Autodesk Inventor part; units mm, degrees
(part 5 of 5)
  arc A2302 (-16.614, -14.2919) -> (-16.722, -14.4863) centre (-15.5907, -14.9875) ccw
  arc A2303 (-16.722, -14.4863) -> (-16.6833, -14.5457) centre (-16.6833, -14.5034) ccw
  arc A2304 (-16.6833, -14.5457) -> (-16.364, -14.4221) centre (-16.6833, -14.0714) ccw
  arc A2305 (-16.364, -14.4221) -> (-15.7284, -13.8044) centre (-25.5328, -4.3522) ccw
  arc A2306 (-15.7284, -13.8044) -> (-15.1286, -13.148) centre (-27.7148, -2.2486) ccw
  arc A2307 (-15.1286, -13.148) -> (-15.136, -12.9408) centre (-15.2436, -13.0484) ccw
  arc A2308 (-15.136, -12.9408) -> (-15.2228, -12.932) centre (-15.1848, -12.9895) ccw
  arc A2309 (-15.2228, -12.932) -> (-15.4687, -13.1078) centre (-12.9519, -16.3686) ccw
  arc A2310 (-15.4687, -13.1078) -> (-15.7663, -13.3595) centre (-12.8053, -16.5585) ccw
  arc A2311 (-15.7663, -13.3595) -> (-16.0961, -13.6818) centre (-9.9901, -19.6001) ccw
  arc A2312 (-8.394, -13.5401) -> (-8.765, -14.0544) centre (-6.9912, -14.9428) ccw
  arc A2313 (-8.765, -14.0544) -> (-8.8769, -14.5817) centre (-7.8107, -14.5324) ccw
  arc A2314 (-8.8769, -14.5817) -> (-8.7186, -15.1214) centre (-7.6904, -14.5268) ccw
  arc A2315 (-8.7186, -15.1214) -> (-8.2954, -15.6725) centre (-6.4085, -13.7855) ccw
  arc A2316 (-8.2954, -15.6725) -> (-7.8135, -16.0761) centre (-5.7719, -13.1489) ccw
  arc A2317 (-7.8135, -16.0761) -> (-7.3942, -16.2454) centre (-7.2343, -15.2456) ccw
  arc A2318 (-7.3942, -16.2454) -> (-6.9318, -16.2189) centre (-7.2235, -15.1778) ccw
  arc A2319 (-6.9318, -16.2189) -> (-6.3068, -15.9905) centre (-8.096, -12.0636) ccw
  arc A2320 (-6.3068, -15.9905) -> (-5.8185, -15.6226) centre (-6.8924, -14.7053) ccw
  arc A2321 (-5.8185, -15.6226) -> (-5.5333, -15.0839) centre (-6.8804, -14.7155) ccw
  arc A2322 (-5.5333, -15.0839) -> (-5.4965, -14.4513) centre (-7.0075, -14.6808) ccw
  arc A2323 (-5.4965, -14.4513) -> (-5.713, -13.8192) centre (-7.3479, -14.7325) ccw
  arc A2324 (-5.713, -13.8192) -> (-6.2117, -13.3188) centre (-6.8518, -14.4553) ccw
  arc A2325 (-6.2117, -13.3188) -> (-6.9584, -13.081) centre (-7.1581, -14.9992) ccw
  arc A2326 (-6.9584, -13.081) -> (-7.7556, -13.1573) centre (-7.1679, -15.0932) ccw
  arc A2327 (-7.7556, -13.1573) -> (-8.394, -13.5401) centre (-7.3105, -14.6235) ccw
  arc A2328 (-6.029, -13.969) -> (-6.4087, -13.5629) centre (-6.8166, -14.325) ccw
  arc A2329 (-5.9189, -14.5767) -> (-6.029, -13.969) centre (-7.1878, -14.4928) ccw
  arc A2330 (-6.1077, -15.2117) -> (-5.9189, -14.5767) centre (-7.4131, -14.4779) ccw
  arc A2331 (-6.549, -15.684) -> (-6.1077, -15.2117) centre (-7.2962, -14.5436) ccw
  arc A2332 (-6.9292, -15.9072) -> (-6.549, -15.684) centre (-9.0119, -11.9251) ccw
  arc A2333 (-7.1687, -15.9661) -> (-6.9292, -15.9072) centre (-7.1687, -15.4493) ccw
  arc A2334 (-7.4082, -15.9072) -> (-7.1687, -15.9661) centre (-7.1687, -15.4493) ccw
  arc A2335 (-7.7884, -15.684) -> (-7.4082, -15.9072) centre (-5.3255, -11.9251) ccw
  arc A2336 (-8.2008, -15.2689) -> (-7.7884, -15.684) centre (-7.0139, -14.5019) ccw
  arc A2337 (-8.392, -14.7361) -> (-8.2008, -15.2689) centre (-7.1547, -14.5929) ccw
  arc A2338 (-8.3266, -14.1792) -> (-8.392, -14.7361) centre (-7.1818, -14.596) ccw
  arc A2339 (-8.0186, -13.6958) -> (-8.3266, -14.1792) centre (-7.0821, -14.6323) ccw
  arc A2340 (-7.6679, -13.4348) -> (-8.0186, -13.6958) centre (-6.9535, -14.7609) ccw
  arc A2341 (-7.296, -13.3246) -> (-7.6679, -13.4348) centre (-7.218, -14.27) ccw
  arc A2342 (-6.8831, -13.3676) -> (-7.296, -13.3246) centre (-7.2037, -14.4426) ccw
  arc A2343 (-6.4087, -13.5629) -> (-6.8831, -13.3676) centre (-7.6118, -15.8109) ccw
  arc A2344 (21.9962, -13.5117) -> (21.6204, -14.3331) centre (23.1058, -14.5159) ccw
  arc A2345 (21.6204, -14.3331) -> (21.7576, -15.2721) centre (23.4017, -14.5523) ccw
  arc A2346 (21.7576, -15.2721) -> (22.3535, -16.0068) centre (23.3891, -14.5579) ccw
  arc A2347 (22.3535, -16.0068) -> (23.2084, -16.2809) centre (23.2084, -14.8107) ccw
  arc A2348 (23.2084, -16.2809) -> (23.7559, -16.143) centre (23.2084, -15.1256) ccw
  arc A2349 (23.7559, -16.143) -> (24.3865, -15.713) centre (22.0269, -12.9297) ccw
  arc A2350 (24.3865, -15.713) -> (24.8982, -15.1775) centre (22.0988, -13.0145) ccw
  arc A2351 (24.8982, -15.1775) -> (25.0563, -14.7143) centre (24.2988, -14.7143) ccw
  arc A2352 (25.0563, -14.7143) -> (25.0229, -14.5369) centre (24.5678, -14.7143) ccw
  arc A2353 (25.0229, -14.5369) -> (24.9054, -14.2755) centre (22.3944, -15.562) ccw
  arc A2354 (24.9054, -14.2755) -> (24.7392, -13.9873) centre (21.9149, -15.8076) ccw
  arc A2355 (24.7392, -13.9873) -> (24.5425, -13.7115) centre (21.7094, -15.9401) ccw
  arc A2356 (24.5425, -13.7115) -> (23.9875, -13.2561) centre (23.2327, -14.7419) ccw
  arc A2357 (23.9875, -13.2561) -> (23.2712, -13.0546) centre (23.1216, -14.9604) ccw
  arc A2358 (23.2712, -13.0546) -> (22.5545, -13.1446) centre (23.1312, -14.8388) ccw
  arc A2359 (22.5545, -13.1446) -> (21.9962, -13.5117) centre (22.9837, -14.4054) ccw
  arc A2360 (24.4962, -14.5242) -> (24.1797, -13.7921) centre (23.2605, -14.6239) ccw
  arc A2361 (24.3036, -15.3024) -> (24.4962, -14.5242) centre (23.2377, -14.6257) ccw
  arc A2362 (23.6761, -15.8191) -> (24.3036, -15.3024) centre (23.2003, -14.602) ccw
  arc A2363 (22.8627, -15.8667) -> (23.6761, -15.8191) centre (23.1962, -14.5915) ccw
  arc A2364 (22.2824, -15.3789) -> (22.8627, -15.8667) centre (23.0863, -15.0116) ccw
  arc A2365 (22.1385, -14.4745) -> (22.2824, -15.3789) centre (23.8394, -14.6676) ccw
  arc A2366 (22.4816, -13.6343) -> (22.1385, -14.4745) centre (23.8009, -14.6632) ccw
  arc A2367 (23.1534, -13.3063) -> (22.4816, -13.6343) centre (23.1534, -14.1582) ccw
  arc A2368 (23.4102, -13.3417) -> (23.1534, -13.3063) centre (23.1534, -14.2548) ccw
  arc A2369 (23.6969, -13.449) -> (23.4102, -13.3417) centre (22.9165, -15.0976) ccw
  arc A2370 (23.9683, -13.6061) -> (23.6969, -13.449) centre (22.885, -15.1641) ccw
  arc A2371 (24.1797, -13.7921) -> (23.9683, -13.6061) centre (23.2607, -14.6237) ccw
  point P0 (0, 0)
  point P1 (50.9531, -6.4169)
  point P2 (50.092, -5.8454)
  point P3 (48.6396, -5.6495)
  point P4 (43.5108, -5.6219)
  point P5 (39.7677, -5.6364)
  point P6 (37.8105, -5.6965)
  point P7 (36.5972, -5.8141)
  point P8 (35.8076, -6.0355)
  point P9 (34.5562, -6.3835)
  point P10 (32.9948, -6.4727)
  point P11 (31.4238, -6.3153)
  point P12 (30.1379, -5.9131)
  point P13 (27.0472, -3.259)
  point P14 (25.8897, 0.6063)
  point P15 (27.0344, 4.4484)
  point P16 (30.1113, 7.0505)
  point P17 (31.4161, 7.4463)
  point P18 (32.9982, 7.603)
  point P19 (34.5626, 7.5186)
  point P20 (35.8076, 7.1795)
  point P21 (36.598, 6.9626)
  point P22 (37.8327, 6.8468)
  point P23 (39.8156, 6.787)
  point P24 (43.5525, 6.7724)
  point P25 (51.1073, 7.8259)
  point P26 (51.8997, 9.0474)
  point P27 (52.1512, 9.8856)
  point P28 (52.0487, 10.8827)
  point P29 (51.4316, 12.9575)
  point P30 (50.503, 16.1693)
  point P31 (50.5853, 17.4879)
  point P32 (51.4074, 18.741)
  point P33 (55.2083, 22.4875)
  point P34 (57.1732, 24.3852)
  point P35 (58.9998, 26.1371)
  point P36 (60.5391, 27.603)
  point P37 (61.2015, 28.2131)
  point P38 (62.1894, 29.2632)
  point P39 (62.7285, 30.2629)
  point P40 (63.0404, 31.6852)
  point P41 (63.3115, 34.5551)
  point P42 (63.4931, 37.4258)
  point P43 (63.4137, 38.7986)
  point P44 (63.0608, 39.6824)
  point P45 (62.3323, 40.4645)
  point P46 (61.7943, 40.78)
  point P47 (61.2117, 40.9238)
  point P48 (60.2699, 40.951)
  point P49 (57.9038, 40.8625)
  point P50 (56.4262, 40.7914)
  point P51 (55.064, 40.7096)
  point P52 (53.9251, 40.6276)
  point P53 (53.4652, 40.5662)
  point P54 (52.6879, 40.2169)
  point P55 (51.3557, 39.1139)
  point P56 (49.183, 37.1068)
  point P57 (44.6444, 32.7271)
  point P58 (42.7401, 30.9041)
  point P59 (41.0144, 29.3026)
  point P60 (39.5441, 27.9774)
  point P61 (39.0671, 27.6446)
  point P62 (38.5752, 27.459)
  point P63 (37.7902, 27.3064)
  point P64 (36.762, 27.1823)
  point P65 (35.4674, 27.0905)
  point P66 (28.6511, 25.0045)
  point P67 (26.8555, 24.1315)
  point P68 (24.7324, 23.1025)
  point P69 (22.6258, 22.0839)
  point P70 (20.8812, 21.2432)
  point P71 (-4.1106, 20.9018)
  point P72 (-5.3285, 21.4718)
  point P73 (-6.4012, 21.9521)
  point P74 (-7.3202, 22.3478)
  point P75 (-7.5227, 22.3891)
  point P76 (-7.6663, 22.4146)
  point P77 (-7.8689, 22.5016)
  point P78 (-8.0891, 22.6255)
  point P79 (-8.2957, 22.7721)
  point P80 (-8.6618, 23.0111)
  point P81 (-10.2026, 23.8217)
  point P82 (-12.033, 24.7645)
  point P83 (-14.1096, 25.8088)
  point P84 (-16.9446, 27.2426)
  point P85 (-18.5176, 28.1127)
  point P86 (-19.4748, 28.7522)
  point P87 (-19.9972, 29.3053)
  point P88 (-20.4506, 30.16)
  point P89 (-20.7879, 31.1801)
  point P90 (-21.1773, 32.913)
  point P91 (-22.0448, 37.3862)
  point P92 (-22.4639, 39.5116)
  point P93 (-22.859, 41.3835)
  point P94 (-23.2124, 42.9637)
  point P95 (-23.3497, 43.3353)
  point P96 (-23.6158, 43.7396)
  point P97 (-23.9597, 44.0911)
  point P98 (-24.6294, 44.6303)
  point P99 (-27.2318, 46.6198)
  point P100 (-28.9487, 47.9049)
  point P101 (-29.8862, 48.5159)
  point P102 (-30.5636, 48.8127)
  point P103 (-31.2169, 48.9127)
  point P104 (-31.7218, 48.8755)
  point P105 (-32.1386, 48.7625)
  point P106 (-32.5186, 48.5551)
  point P107 (-32.9118, 48.231)
  point P108 (-33.7482, 47.2048)
  point P109 (-35.3625, 44.5463)
  point P110 (-36.924, 41.8255)
  point P111 (-37.3199, 40.7523)
  point P112 (-37.3294, 40.2564)
  point P113 (-36.8969, 37.6163)
  point P114 (-36.3581, 34.5397)
  point P115 (-35.6931, 31.0149)
  point P116 (-34.8694, 26.6834)
  point P117 (-34.3851, 23.8802)
  point P118 (-34.0925, 21.9108)
  point P119 (-34.155, 21.3608)
  point P120 (-34.3185, 21.062)
  point P121 (-34.6814, 20.6027)
  point P122 (-35.1373, 20.0934)
  point P123 (-35.6353, 19.6)
  point P124 (-47.0034, 18.4056)
  point P125 (-51.1447, 18.4014)
  point P126 (-55.2197, 18.4031)
  point P127 (-58.7387, 18.4096)
  point P128 (-60.7691, 18.4215)
  point P129 (-63.1356, 18.4303)
  point P130 (-64.0239, 18.3685)
  point P131 (-64.5589, 18.193)
  point P132 (-65.0451, 17.8304)
  point P133 (-65.3966, 17.3849)
  point P134 (-65.5766, 16.9262)
  point P135 (-65.6529, 16.2301)
  point P136 (-65.6695, 14.6996)
  point P137 (-65.6518, 13.7068)
  point P138 (-65.5983, 12.7955)
  point P139 (-65.5226, 12.0428)
  point P140 (-65.4277, 11.7416)
  point P141 (-65.2326, 11.5002)
  point P142 (-64.683, 11.0546)
  point P143 (-63.996, 10.5482)
  point P144 (-63.2287, 10.0344)
  point P145 (-62.3944, 9.4689)
  point P146 (-61.7482, 8.9601)
  point P147 (-61.2933, 8.5231)
  point P148 (-61.1189, 8.2094)
  point P149 (-60.9236, 6.7099)
  point P150 (-60.9654, 0.2597)
  point P151 (-61.0492, -6.4223)
  point P152 (-61.2783, -7.2762)
  point P153 (-61.5015, -7.5553)
  point P154 (-62.0441, -8.0177)
  point P155 (-62.7195, -8.5338)
  point P156 (-63.4625, -9.0436)
  point P157 (-64.1955, -9.5449)
  point P158 (-64.8377, -10.0333)
  point P159 (-65.3508, -10.4676)
  point P160 (-65.5076, -10.694)
  point P161 (-65.5713, -10.9747)
  point P162 (-65.6219, -11.7177)
  point P163 (-65.6576, -12.609)
  point P164 (-65.6695, -13.5856)
  point P165 (-65.6527, -15.0785)
  point P166 (-65.5769, -15.7726)
  point P167 (-65.4007, -16.2293)
  point P168 (-65.061, -16.664)
  point P169 (-35.56, -18.5257)
  point P170 (-35.0417, -19.0492)
  point P171 (-34.5802, -19.5857)
  point P172 (-34.2239, -20.0672)
  point P173 (-34.0855, -20.3742)
  point P174 (-34.0594, -21.0488)
  point P175 (-34.6127, -24.2087)
  point P176 (-35.4855, -28.8682)
  point P177 (-37.0712, -36.9536)
  point P178 (-37.2096, -37.7513)
  point P179 (-37.3057, -38.5299)
  point P180 (-37.3541, -39.1971)
  point P181 (-37.3261, -39.5707)
  point P182 (-36.9138, -40.6825)
  point P183 (-35.2402, -43.5792)
  point P184 (-33.5006, -46.4468)
  point P185 (-32.7638, -47.2701)
  point P186 (-32.1559, -47.5931)
  point P187 (-31.38, -47.7432)
  point P188 (-30.579, -47.7064)
  point P189 (-29.8958, -47.4767)
  point P190 (-29.5663, -47.2708)
  point P191 (-28.7959, -46.6994)
  point P192 (-27.8869, -46.0031)
  point P193 (-26.9121, -45.232)
  point P194 (-25.9442, -44.4614)
  point P195 (-25.0535, -43.7647)
  point P196 (-24.304, -43.1885)
  point P197 (-24.0171, -42.9901)
  point P198 (-23.5257, -42.4562)
  point P199 (-23.1456, -41.4944)
  dimension "d2" = 130.09
  constraints: 4746 point on circle, 2372 centre point, 200 end point
  measures "d2" horizontal distance of point (-66.161, -14.456) point (63.929, -37.224)
extrude "Extrusion1" add sketch "Sketch1" along normal blind 3 contours A249 A250 A251 A252 A253 A254 A255 A256 A257 A258 A259 A260 A261 A262 A263 A264 A265 A266 A267 A268 A269 A270 A271 A272 A273 A274 A275 L22 L23 L24 L25 A276 A277 A278 A279 L26 L27 A280 A281 A282 A283 A284 A285 A286 A287 A288 A289 A290 A291 A292 A293 A294 A295 A296 A297 A298 A299 A300 A301 A302 A303 A304 A305 A306 A307 A308 A309 A310 A311 A312 A313 A314 A315 A316 A317 A318 A319 L28 L29 A320 A321 A322 A323 A324 A325 A326 A327 A328 A329 A330 A331 A332 A333 A334 A335 A336 A337 A338 A339 A340 A341 A342 A343 L30 L31 A344 A345 A346 A347 A348 A349 A350 A351 A352 A353 A354 A355 A356 A357 A358 A359 A360 A361 A362 A363 A364 A365 A366 A367 A368 A369 A370 A371 A372 A373 A374 A375 A376 A377 A378 A379 A380 A381 A382 A383 L32 L33 L34 L35 L36 L37 A384 A385 A386 A387 A388 A389 A390 A391 A392 A393 A394 A395 A396 A397 A398 A399 A400 A401 A402 A403 A404 A405 A406 A407 A408 A409 A410 A411 A412 A413 A414 A415 A416 A417 A418 A419 A420 A421 A422 A423 L38 L39 L40 L41 A424 A425 A426 A427 A428 A429 A430 A431 A432 A433 A434 A435 A436 A437 A438 A439 A440 A441 A442 A443 A444 A445 A446 A447 A448 A449 A450 A451 A452 A453 A454 A455 A456 A457 A458 A459 A460 A461 A462 A463 A464 A465 A466 A467 L42 L43 A468 A469 A470 A471 A472 A473 A474 A475 A476 A477 A478 A479 A480 A481 A482 A483 A484 A485 A486 A487 A488 A489 A490 A491 A248
sketch "Sketch2" plane through (0, 3, 0) normal (0, 1, 0) x (1, 0, 0)
  circle A0 centre (-23.6086, 14.5288) radius 4.9273
  circle A1 centre (6.6771, 14.5288) radius 4.6599
  circle A2 centre (6.6771, -16.1286) radius 5.0518
  circle A3 centre (-23.6086, -16.1286) radius 5.1742
  point P0 (0, 0)
  constraints: 4 centre point
extrude "Extrusion2" add sketch "Sketch2" against normal blind 3
sketch "Sketch3" plane through (0, 3, 0) normal (0, 1, 0) x (1, 0, 0)
  circle A0 centre (-23.2436, 14.6296) radius 1.6
  circle A1 centre (7.2564, 14.6296) radius 1.6
  circle A2 centre (7.6901, -15.8704) radius 1.6
  circle A3 centre (-22.8099, -15.8704) radius 1.6
  arc A4 (-25.8897, -0.6058) -> (-27.0473, 3.2592) centre (-32.9695, -0.6204) ccw projected
  line L0 (-32.9695, -0.6204) -> (10.6901, -0.6204)
  line L1 (-15.6666, -0.6204) -> (-0.3205, -0.6204)
  line L2 (-7.9936, -0.6204) -> (-7.9936, 21.9698)
  line L3 (-7.9936, -0.6204) -> (7.2564, -0.6204)
  point P0 (0, 0)
  dimension "d5" = 3.2
  dimension "d6" = 3.2
  dimension "d7" = 3.2
  dimension "d8" = 3.2
  dimension "d9" = 30.5
  dimension "d10" = 30.5
  dimension "d11" = 30.5
  dimension "d12" = 30.5
  dimension "d13" = 15.25
  dimension "d14" = 15.25
  dimension "d17" = 90
  dimension "d18" = 15.25
  dimension "d19" = 15.25
  dimension "d20" = 15.25
  constraints: 8 end point, 4 centre point, 3 point on line, 1 horizontal, 1 midpoint, 1 vertical
  measures "d5" diameter of A0
  measures "d6" diameter of A1
  measures "d7" diameter of A2
  measures "d8" diameter of A3
  measures "d9" distance of A1.centre A0.centre
  measures "d10" vertical distance of A3.centre A0.centre
  measures "d11" distance of A2.centre A3.centre
  measures "d12" vertical distance of A1.centre A2.centre
  measures "d13" distance from line of A0.centre L0
  measures "d14" distance from line of A1.centre L0
  measures "d17" angle of L0 L2
  measures "d18" distance of L2.start L3.end
  measures "d19" distance from line of L3.end L2
  measures "d20" distance from line of A1.centre L2
extrude "Extrusion3" cut sketch "Sketch3" against normal blind 3
sketch "Sketch4" plane through (0, 3, 0) normal (0, 1, 0) x (1, 0, 0)
  circle A0 centre (29.8495, 38.2698) radius 1.5
  circle A1 centre (-55.9919, 32.2964) radius 1.5
  circle A2 centre (-55.9919, -33.39) radius 1.5
  point P0 (0, 0)
  dimension "d23" = 3
  dimension "d24" = 3
  dimension "d25" = 3
  constraints: 3 centre point
  measures "d23" diameter of A0
  measures "d24" diameter of A1
  measures "d25" diameter of A2
extrude "Extrusion4" cut sketch "Sketch4" against normal blind 3
sketch "Sketch5" plane through (0, 3, 0) normal (0, 1, 0) x (1, 0, 0)
  arc A0 (31.3101, 37.9283) -> (31.3401, 38.4374) centre (29.8495, 38.2698) ccw projected
  circle A1 centre (29.8495, 38.2698) radius 1.5
  arc A2 (-54.5163, 32.0268) -> (-54.5234, 32.6024) centre (-55.9919, 32.2964) ccw projected
  circle A3 centre (-55.9919, 32.2964) radius 1.5
  arc A4 (-54.5453, -33.7867) -> (-54.495, -33.2937) centre (-55.9919, -33.39) ccw projected
  circle A5 centre (-55.9919, -33.39) radius 1.5
  circle A6 centre (-55.9919, -33.39) radius 4.0652
  circle A7 centre (-55.9919, 32.2964) radius 3.7909
  circle A8 centre (29.8495, 38.2698) radius 4.0357
  arc A9 (-30.1113, -7.0505) -> (-27.0344, -4.4484) centre (-32.9692, -0.5508) ccw projected
  line L0 (-32.9692, -0.5508) -> (85.1514, -0.5508)
  arc A10 (31.3401, -39.5391) -> (31.3101, -39.03) centre (29.8495, -39.3715) ccw
  circle A11 centre (29.8495, -39.3715) radius 1.5
  circle A12 centre (29.8495, -39.3715) radius 4.0357
  point P0 (0, 0)
  point P1 (-54.5234, 32.6024)
  point P2 (31.3401, 38.4374)
  point P3 (-54.495, -33.2937)
  constraints: 9 centre point, 8 coincident, 5 symmetric about line, 2 end point, 2 point on circle, 1 horizontal, 3 other
extrude "Extrusion5" add sketch "Sketch5" against normal blind 3
sketch "Sketch6" plane through (0, 3, 0) normal (0, 1, 0) x (1, 0, 0)
  arc A0 (-27.0344, -4.4484) -> (-25.8897, -0.6058) centre (-32.8637, -0.6201) ccw projected
  line L0 (-32.8637, -0.6201) -> (101.6053, -0.6201)
  circle A1 centre (-47.7405, 9.4799) radius 1.5
  circle A2 centre (-47.7405, -10.7202) radius 1.5
  circle A3 centre (-47.7405, 9.4799) radius 2.5
  circle A4 centre (-47.7405, -10.7202) radius 2.5
  line L1 (-43.5524, -6.7724) -> (-50.3374, -6.7724) projected
  arc A5 (-48.6396, 5.6495) -> (-43.5108, 5.6219) centre (-43.5104, 481.9367) ccw projected
  line L2 (-48.6396, 5.6495) -> (-43.5108, 5.6219)
  point P0 (0, 0)
  point P1 (-46.9449, -6.7724)
  dimension "d31" = 3
  dimension "d32" = 5
  dimension "d33" = 5
  dimension "d38" = 3.9478
  dimension "d39" = 3.8352
  constraints: 4 centre point, 4 end point, 2 coincident, 1 horizontal, 1 midpoint, 1 symmetric about line, 1 other
  measures "d31" diameter of A1
  measures "d32" diameter of A3
  measures "d33" diameter of A4
  measures "d38" vertical distance of point (-46.945, -6.772) A2.centre
  measures "d39" distance from line of L2 A1.centre
extrude "Extrusion6" add sketch "Sketch6" against normal blind 3 contours A3 | A4
sketch "Sketch7" plane through (0, 3, 0) normal (0, 1, 0) x (1, 0, 0)
  arc A0 (-46.7804, -11.8727) -> (-49.1973, -11.0777) centre (-47.7405, -10.7202) ccw projected
  circle A1 centre (-47.7405, -10.7202) radius 1.5
  point P0 (0, 0)
  point P1 (-49.1973, -11.0777)
  constraints: 1 centre point, 1 coincident
extrude "Extrusion7" cut sketch "Sketch7" against normal blind 3
sketch "Sketch8" plane through (0, 3, 0) normal (0, 1, 0) x (1, 0, 0)
  line L0 (17.2292, 11.9933) -> (18.6119, 7.4214)
  line L1 (18.6119, 7.4214) -> (20.9091, 5.9717)
  line L2 (20.9091, 5.9717) -> (27.6415, 12.1528)
  line L3 (26.4888, 13.4084) -> (28.7346, 10.9622) projected
  arc A0 (26.1413, 13.6754) -> (24.322, 15.5252) centre (-95.7981, -104.4298) ccw projected
  line L4 (25.34, 14.4971) -> (18.2939, 10.9088)
  line L5 (25.34, 14.4971) -> (27.6415, 12.1528)
  line L6 (17.2292, 11.9933) -> (24.322, 15.5252)
  line L7 (18.2939, 10.9088) -> (19.1309, 12.9403)
  point P0 (0, 0)
  constraints: 14 end point, 2 point on line, 1 point on circle, 1 tangent
extrude "Extrusion8" cut sketch "Sketch8" against normal blind 3 contours L6 L7 L4 L5 L2 L1 L0
sketch "Sketch9" plane through (0, 3, 0) normal (0, 1, 0) x (1, 0, 0)
  arc A0 (-27.0344, -4.4484) -> (-25.8897, -0.6058) centre (-32.8637, -0.6201) ccw projected
  line L0 (-32.8637, -0.6201) -> (88.4587, -0.6201)
  circle A1 centre (59.9231, -14.6201) radius 1.5
  circle A2 centre (59.9231, 13.3799) radius 1.5
  circle A3 centre (37.0306, 9.3799) radius 1.5
  circle A4 centre (37.0306, -10.6201) radius 1.5
  circle A5 centre (37.0306, 9.3799) radius 4.2001
  circle A6 centre (59.9231, 13.3799) radius 2.8139
  circle A7 centre (59.9231, -14.6201) radius 3.1887
  circle A8 centre (37.0306, -10.6201) radius 3.5086
  point P0 (0, 0)
  dimension "d42" = 3
  dimension "d43" = 3
  dimension "d44" = 3
  dimension "d45" = 3
  dimension "d46" = 14
  dimension "d47" = 14
  dimension "d48" = 10
  dimension "d49" = 10
  dimension "d50" = 22.8925
  constraints: 8 centre point, 4 coincident, 2 end point, 1 horizontal
  measures "d42" diameter of A1
  measures "d43" diameter of A2
  measures "d44" diameter of A3
  measures "d45" diameter of A4
  measures "d46" distance from line of A2.centre L0
  measures "d47" distance from line of L0 A1.centre
  measures "d48" distance from line of L0 A3.centre
  measures "d49" distance from line of L0 A4.centre
  measures "d50" horizontal distance of A2.centre A3.centre
extrude "Extrusion9" add sketch "Sketch9" against normal blind 3
sketch "Sketch10" plane through (0, 3, 0) normal (0, 1, 0) x (1, 0, 0)
  arc A0 (59.6137, -16.0879) -> (58.9632, -15.7728) centre (59.9231, -14.6201) ccw projected
  circle A1 centre (59.9231, -14.6201) radius 1.5
  point P0 (0, 0)
  point P1 (58.9632, -15.7728)
  point P2 (59.6137, -16.0879)
  constraints: 1 centre point, 1 coincident
extrude "Extrusion10" cut sketch "Sketch10" against normal blind 3
sketch "Sketch11" plane through (0, 3, 0) normal (0, 1, 0) x (1, 0, 0)
  circle A0 centre (53.4541, -0.5633) radius 2
  circle A1 centre (53.4541, -0.5633) radius 4.9271
  point P0 (0, 0)
  dimension "d55" = 4
  constraints: 2 centre point, 1 coincident
  measures "d55" diameter of A0
extrude "Extrusion11" add sketch "Sketch11" against normal blind 3
sketch "Sketch12" plane through (0, 3, 0) normal (0, 1, 0) x (1, 0, 0)
  circle A0 centre (50.9743, 12.0462) radius 2.3423
  circle A1 centre (46.9866, 4.4135) radius 2.5247
  circle A2 centre (47.1514, -5.6618) radius 3.8714
  circle A3 centre (51.2732, -13.4167) radius 2.3203
  point P0 (0, 0)
  constraints: 4 centre point
extrude "Extrusion12" add sketch "Sketch12" against normal blind 3
sketch "Sketch13" plane through (0, 3, 0) normal (0, 1, 0) x (1, 0, 0)
  arc A0 (-30.1113, -7.0505) -> (-27.0344, -4.4484) centre (-32.9692, -0.5508) ccw projected
  line L0 (-32.9692, -0.5508) -> (82.6738, -0.5508)
  circle A1 centre (47.0233, 4.4492) radius 1.05
  arc A2 (61.0492, 6.4223) -> (60.9654, -0.2597) centre (1550.8386, -15.5871) ccw projected
  line L1 (61.0492, 6.4223) -> (60.9654, -0.2597)
  circle A3 centre (51.0233, 12.4492) radius 1.05
  circle A4 centre (47.0233, -5.5508) radius 1.05
  circle A5 centre (51.0233, -13.5508) radius 1.05
  point P0 (0, 0)
  dimension "d60" = 2.1
  dimension "d61" = 5
  dimension "d62" = 14
  dimension "d63" = 2.1
  dimension "d64" = 8
  dimension "d65" = 4
  constraints: 4 centre point, 4 end point, 2 symmetric about line, 1 horizontal, 2 other
  measures "d60" diameter of A1
  measures "d61" distance from line of L0 A1.centre
  measures "d62" distance from line of L1 A1.centre
  measures "d63" diameter of A3
  measures "d64" vertical distance of A3.centre A1.centre
  measures "d65" horizontal distance of A1.centre A3.centre
extrude "Extrusion13" cut sketch "Sketch13" against normal blind 3 contours A1 | A3 | A4 | A5
sketch "Sketch14" plane through (0, 3, 0) normal (0, 1, 0) x (1, 0, 0)
  circle A0 centre (-22.8099, -15.8704) radius 1.6 projected
  circle A1 centre (7.2564, 14.6296) radius 1.6 projected
  line L0 (-22.8099, -15.8704) -> (7.2564, 14.6296)
  circle A2 centre (-23.2436, 14.6296) radius 1.6 projected
  circle A3 centre (7.6901, -15.8704) radius 1.6 projected
  line L1 (-23.2436, 14.6296) -> (7.6901, -15.8704)
  circle A4 centre (-23.2436, 14.6296) radius 2.5
  circle A5 centre (7.2564, 14.6296) radius 2.5
  circle A6 centre (7.6901, -15.8704) radius 2.5
  circle A7 centre (-22.8099, -15.8704) radius 2.5
  circle A8 centre (-23.2436, 14.6296) radius 1.6
  circle A9 centre (7.2564, 14.6296) radius 1.6
  circle A10 centre (7.6901, -15.8704) radius 1.6
  circle A11 centre (-22.8099, -15.8704) radius 1.6
  circle A12 centre (-23.2436, 14.6296) radius 1.6
  circle A13 centre (7.2564, 14.6296) radius 1.6
  circle A14 centre (7.6901, -15.8704) radius 1.6
  circle A15 centre (-22.8099, -15.8704) radius 1.5
  point P0 (0, 0)
  dimension "d68" = 5
  dimension "d69" = 5
  dimension "d70" = 5
  dimension "d71" = 5
  constraints: 12 centre point, 11 coincident, 7 concentric, 4 end point, 1 point on line
  measures "d68" diameter of A4
  measures "d69" diameter of A5
  measures "d70" diameter of A6
  measures "d71" diameter of A7
extrude "Extrusion14" add sketch "Sketch14" along normal blind 1 contours A7 | A4 | A5 | A6
sketch "Sketch15" plane through (0, 3, 0) normal (0, 1, 0) x (1, 0, 0)
  circle A0 centre (-23.2436, 14.6296) radius 1.6 projected
  circle A1 centre (7.6901, -15.8704) radius 1.6 projected
  line L0 (-23.2436, 14.6296) -> (7.6901, -15.8704)
  circle A2 centre (-22.8099, -15.8704) radius 1.6 projected
  circle A3 centre (7.2564, 14.6296) radius 1.6 projected
  line L1 (-22.8099, -15.8704) -> (7.2564, 14.6296)
  line L2 (-7.7767, -0.6204) -> (-7.7767, 19.3796)
  line L3 (-7.7767, 19.3796) -> (3.7233, 19.3796)
  line L4 (3.7233, 19.3796) -> (3.7233, -20.6204)
  line L5 (3.7233, -20.6204) -> (-19.2767, -20.6204)
  line L6 (-19.2767, -20.6204) -> (-19.2767, 19.3796)
  line L7 (-19.2767, 19.3796) -> (-7.7767, 19.3796)
  point P0 (0, 0)
  dimension "d74" = 20
  dimension "d75" = 11.5
  dimension "d76" = 40
  dimension "d77" = 23
  constraints: 16 end point, 4 perpendicular, 1 horizontal, 1 midpoint, 1 vertical
  measures "d74" distance of L2.start L2.end
  measures "d75" distance of L2.end L3.end
  measures "d76" distance of L3.end L4.end
  measures "d77" distance of L4.end L5.end
extrude "Extrusion15" cut sketch "Sketch15" against normal blind 0.5 contours L6 L7 L2 L0 | L0 L1 L6 | L1 L4 L0 | L0 L4 L5 L6 L1 | L2 L3 L4 L1
sketch "Sketch17" plane through (0, 2.5, 0) normal (0, 1, 0) x (1, 0, 0)
  arc A0 (-27.0344, -4.4484) -> (-25.8897, -0.6058) centre (-32.8637, -0.6201) ccw projected
  line L0 (-32.8637, -0.6201) -> (36.5369, -0.6201)
  line L1 (-19.2767, -20.4716) -> (-19.2767, 19.3308) projected
  line L2 (-19.2767, -0.5704) -> (-17.2774, -0.6201)
  line L3 (-17.0783, -19.4145) -> (0.9872, -19.4145) projected
  line L4 (-17.2774, -0.6201) -> (-17.0783, -19.4145)
  line L5 (-19.2767, 19.3308) -> (-17.075, 18.264) projected
  line L6 (-17.2774, -0.6201) -> (-17.075, 18.264)
  line L7 (3.7233, 19.3796) -> (3.7233, -20.6204) projected
  line L8 (3.7233, -0.6204) -> (1.7233, -0.6201)
  line L9 (1.7233, -0.6201) -> (1.7253, 18.6194)
  line L10 (0.9918, 18.264) -> (3.2943, 19.3796) projected
  line L11 (1.7233, -0.6201) -> (1.7233, -19.765)
  line L12 (3.5196, -20.6204) -> (0.9872, -19.4145) projected
  line L13 (-17.075, 18.264) -> (1.728, 44.6098)
  line L14 (1.728, 44.6098) -> (1.7253, 18.6194)
  line L15 (1.7233, -19.765) -> (1.7195, -36.2978)
  line L16 (1.7195, -36.2978) -> (-17.0783, -19.4145)
  point P0 (0, 0)
  dimension "d80" = 2
  dimension "d81" = 2
  constraints: 22 end point, 4 point on line, 2 midpoint, 1 horizontal, 1 perpendicular, 1 vertical
  measures "d80" distance of L2.start L2.end
  measures "d81" distance of L8.start L8.end
extrude "Extrusion16" cut sketch "Sketch17" against normal blind 1.5 contours L6 L13 L14 L9 L0 | L0 L11 L12 L3 L4 | L3 L12 L15 L16
sketch "Sketch23" plane through (0, 3, 0) normal (0, 1, 0) x (1, 0, 0)
  line L0 (3.5196, -20.6204) -> (4.1106, -20.9018) projected
  line L1 (3.7291, -20.7201) -> (-8.0702, -20.7201)
  line L2 (-8.0702, -20.7201) -> (-8.0702, 34.9354)
  line L3 (-8.0702, 34.9354) -> (3.7291, 34.9354)
  line L4 (3.7291, 34.9354) -> (3.7291, -20.7201)
  point P0 (0, 0)
  constraints: 8 end point, 2 parallel, 1 horizontal, 1 perpendicular, 1 point on line
extrude "Extrusion22" cut sketch "Sketch23" against normal blind 0.5
sketch "Sketch25" plane through (0, 3, 0) normal (0, 1, 0) x (1, 0, 0)
  line L0 (-17.0783, -19.4145) -> (-19.2767, -20.4716) projected
  line L1 (9.9588, 22.6088) -> (0.9918, 18.264) projected
  line L2 (-17.0783, -19.4145) -> (0.9918, -19.4145)
  line L3 (0.9918, -19.4145) -> (0.9918, 18.264)
  line L4 (0.9918, 18.264) -> (-17.0783, 18.264)
  line L5 (-17.0783, 18.264) -> (-17.0783, -19.4145)
  line L6 (0.9918, 18.264) -> (3.7291, 19.5903)
  line L7 (3.7291, 19.5903) -> (3.7291, -20.7201) projected
  line L8 (3.7291, 19.5903) -> (3.7291, -20.7201)
  line L9 (3.7291, -20.7201) -> (0.9918, -19.4145)
  line L10 (-17.0783, -19.4145) -> (-19.2767, -20.4716)
  line L11 (-19.2767, -20.4716) -> (-19.2767, 19.3308) projected
  line L12 (-19.2767, -20.4716) -> (-19.2767, 19.3308)
  line L13 (-19.2767, 19.3308) -> (-17.0783, 18.264)
  point P0 (0, 0)
  constraints: 20 end point, 3 equal length, 1 horizontal, 1 perpendicular, 1 point on line, 1 vertical
extrude "Extrusion24" add sketch "Sketch25" against normal blind 3
sketch "Sketch26" plane through (0, 3, 0) normal (0, 1, 0) x (1, 0, 0)
  arc A0 (22.7174, 39.7245) -> (21.9043, 35.5673) centre (511.1801, -57.9702) ccw projected
  line L0 (21.9043, 35.5673) -> (50.154, 183.336)
  arc A1 (37.0712, 36.9536) -> (35.4855, 28.8679) centre (2745.9567, -498.4883) ccw projected
  line L1 (35.4855, 28.8679) -> (64.9873, 180.4994)
  circle A2 centre (57.8174, 183.336) radius 7.7106
  line L2 (21.9043, 35.5673) -> (35.4855, 28.8679)
  arc A3 (-30.1113, -7.0505) -> (-27.0344, -4.4484) centre (-32.9692, -0.5508) ccw projected
  line L3 (-32.9692, -0.5508) -> (-8.5446, -0.5508)
  arc A4 (21.9043, -36.669) -> (22.7174, -40.8262) centre (511.1801, 56.8685) ccw
  line L4 (21.9043, -36.669) -> (50.154, -184.4377)
  arc A5 (35.4855, -29.9696) -> (37.0712, -38.0553) centre (2745.9567, 497.3866) ccw
  line L5 (35.4855, -29.9696) -> (64.9873, -181.6011)
  circle A6 centre (57.8174, -184.4377) radius 7.7106
  line L6 (21.9043, -36.669) -> (35.4855, -29.9696)
  arc A7 (-47.8615, 34.6906) -> (-43.2688, 30.2663) centre (1782.7173, 1930.371) ccw projected
  line L7 (-43.2688, 30.2663) -> (-161.509, 151.4367)
  arc A8 (-52.5304, 18.7828) -> (-58.694, 24.7351) centre (-3130.1027, -3161.8952) ccw projected
  line L8 (-52.5304, 18.7828) -> (-171.9931, 141.2061)
  line L9 (-171.9931, 141.2061) -> (-161.509, 151.4367)
  circle A9 centre (-166.751, 146.3214) radius 7.3243
  line L10 (-52.5304, 18.7828) -> (-43.2688, 30.2663)
  arc A10 (-43.2688, 30.2663) -> (-41.045, 28.1667) centre (76.8371, 155.2473) ccw projected
  arc A11 (-43.2688, -31.368) -> (-47.8615, -35.7923) centre (1782.7173, -1931.4727) ccw
  line L11 (-43.2688, -31.368) -> (-161.509, -152.5384)
  arc A12 (-58.694, -25.8368) -> (-52.5304, -19.8845) centre (-3130.1027, 3160.7935) ccw
  line L12 (-52.5304, -19.8845) -> (-171.9931, -142.3078)
  line L13 (-171.9931, -142.3078) -> (-161.509, -152.5384)
  circle A13 centre (-166.751, -147.4231) radius 7.3243
  line L14 (-52.5304, -19.8845) -> (-43.2688, -31.368)
  arc A14 (-41.045, -29.2684) -> (-43.2688, -31.368) centre (76.8371, -156.349) ccw
  point P0 (0, 0)
  point P1 (50.1102, 183.1069)
  point P2 (50.1102, -184.2086)
  point P3 (-171.9931, 141.2061)
  constraints: 30 end point, 22 symmetric about line, 14 point on circle, 5 centre point, 3 horizontal, 2 point on line, 2 tangent, 1 midpoint, 1 parallel, 17 other
extrude "Extrusion25" add sketch "Sketch26" against normal blind 3
sketch "Sketch27" plane through (0, 3, 0) normal (0, 1, 0) x (1, 0, 0)
  line L0 (2.5588, 7.6763) -> (14.7911, 16.4959)
  line L1 (14.7911, 16.4959) -> (26.1866, 23.029)
  line L2 (26.1866, 23.029) -> (31.7397, 7.6763)
  line L3 (31.7397, 7.6763) -> (31.7397, -17.8026)
  line L4 (31.7397, -17.8026) -> (20.4889, -25.9145)
  line L5 (20.4889, -25.9145) -> (9.9183, -11.2536)
  line L6 (9.9183, -11.2536) -> (0.7077, -9.7451)
  line L7 (0.7077, -9.7451) -> (2.5588, 7.6763)
  line L8 (-42.9641, 19.7461) -> (-27.8918, 15.4972)
  line L9 (-27.8918, 15.4972) -> (-24.9576, 4.8081)
  line L10 (-24.9576, 4.8081) -> (-21.4242, -8.0633)
  line L11 (-21.4242, -8.0633) -> (-31.9676, -20.8613)
  line L12 (-31.9676, -20.8613) -> (-41.2126, -21.8585)
  line L13 (-41.2126, -21.8585) -> (-42.5193, -9.7451)
  line L14 (-43.5524, -6.7724) -> (-50.3374, -6.7724) projected
  line L15 (-42.5193, -9.7451) -> (-50.3374, -6.7724)
  arc A0 (-50.9531, 6.4169) -> (-50.092, 5.8454) centre (-49.6841, 7.3946) ccw projected
  line L16 (-50.3374, -6.7724) -> (-50.092, 5.8454)
  line L17 (-50.092, 5.8454) -> (-45.0482, 7.23)
  line L18 (-45.0482, 7.23) -> (-42.9641, 19.7461)
  line L19 (-51.6087, 11.162) -> (-52.3994, 8.8937) projected
  line L20 (-52.3994, 8.8937) -> (-52.1512, -9.8856)
  line L21 (-52.1512, -9.8856) -> (-50.3374, -6.7724)
  line L22 (-52.3994, 8.8937) -> (-51.8428, 7.8155) projected
  line L23 (-52.3994, 8.8937) -> (-50.8258, 8.5185)
  line L24 (-50.8258, 8.5185) -> (-50.092, 5.8454)
  point P0 (0, 0)
  constraints: 44 end point, 3 perpendicular, 1 parallel, 1 point on line, 1 vertical
extrude "Extrusion26" add sketch "Sketch27" against normal blind 3
sketch "Sketch28" plane through (0, 3, 0) normal (0, 1, 0) x (1, 0, 0)
  line L0 (64.4526, 17.2724) -> (36.8852, 17.2724) projected
  line L1 (64.4526, 17.2724) -> (-59.384, 17.2724)
  ellipse E0 centre (47.4324, -18.7075) end of major axis (77.2601, -18.6604) minor radius 0.3026 (58.7385, -18.4096) -> (51.1447, -18.4014) ccw projected
  line L2 (-97.9059, -18.0059) -> (-234.3365, -155.642)
  line L3 (-234.3365, -155.642) -> (58.1177, -259.2673)
  line L4 (58.1177, -259.2673) -> (143.832, -191.9895)
  line L5 (143.832, -191.9895) -> (134.5518, -61.2932)
  line L6 (134.5518, -61.2932) -> (47.4324, -18.7075)
  line L7 (-59.384, 17.2724) -> (-204.9491, 60.8962)
  line L8 (-204.9491, 60.8962) -> (-214.241, 191.7564)
  line L9 (-214.241, 191.7564) -> (126.045, 241.0869)
  line L10 (126.045, 241.0869) -> (186.3663, 60.8962)
  line L11 (186.3663, 60.8962) -> (47.4324, 17.2724)
  line L12 (36.8936, -18.4229) -> (47.0034, -18.4056) projected
  line L13 (62.5866, -18.5283) -> (-85.9025, -18.5283)
  line L14 (-98.4238, -18.5283) -> (-85.9025, -18.5283)
  line L15 (47.4324, -18.7075) -> (62.5866, -18.5283)
  point P0 (0, 0)
  constraints: 28 end point, 3 horizontal, 2 point on line, 1 other
extrude "Extrusion27" cut sketch "Sketch28" against normal blind 10
sketch "Sketch29" plane through (0, 3, 0) normal (0, 1, 0) x (1, 0, 0)
  line L0 (64.4526, 17.2724) -> (-51.0694, 17.2724) projected
  line L1 (64.4526, 17.2724) -> (-176.3986, 17.2724)
  arc A0 (-51.2113, -18.5283) -> (-50.5853, -17.4879) centre (-54.0351, -16.1207) ccw projected
  line L2 (-51.2113, -18.5283) -> (-37.033, -18.5283)
  line L3 (-37.033, -18.5283) -> (-176.3986, -18.5283)
  line L4 (-176.3986, 17.2724) -> (-176.3986, -18.5283)
  line L5 (-47.18, -18.5283) -> (-50.5853, -10.3326)
  line L6 (-50.5853, -10.3326) -> (-50.5853, 0)
  line L7 (-50.5853, 0) -> (-50.1722, 9.8647)
  line L8 (-50.1722, 9.8647) -> (-49.5898, 17.2724)
  point P0 (0, 0)
  point P1 (-51.0694, 17.2724)
  constraints: 16 end point, 3 point on line, 2 horizontal, 2 vertical
extrude "Extrusion28" add sketch "Sketch29" against normal blind 3
fillet "Fillet1" radius 3 2 edges at (-176.3986, 1.5, 18.5283) (-176.3986, 1.5, -17.2724)
body "Solid1"
